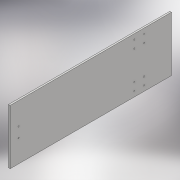
# Autodesk Inventor part: 内层17cm板
Saved by Autodesk Inventor 2017 (Build 210142000, 142)
## iProperties
Part Number: 内层17cm板
Material: 常规
Document SubType Name: 钣金
Designer: PANDA
Density: 1 g/cm^3
Sheet Metal Rule: 默认_mm
Appearance: 默认
Author: PANDA
Autodesk Inventor part; units mm, degrees
ref_plane "YZ Plane" through (0, 0, 0) normal (1, 0, 0) x (0, 1, 0)
ref_plane "XZ Plane" through (0, 0, 0) normal (0, 1, 0) x (-1, 0, 0)
ref_plane "XY Plane" through (0, 0, 0) normal (0, 0, 1) x (1, 0, 0)
sketch "草图8" plane through (0, 0, 0) normal (1, 0, 0) x (0, 1, 0)
  line L0 (250, 85) -> (-250, 85)
  line L1 (-250, 85) -> (-250, -85)
  line L2 (-250, -85) -> (250, -85)
  line L3 (250, -85) -> (250, 85)
  point P0 (0, 0)
  dimension "d22" = 500
  dimension "d23" = 170
  constraints: 8 end point, 2 parallel, 1 horizontal, 1 perpendicular
  measures "d22" distance of L2.end L1.end
  measures "d23" distance of L1.end L0.end
extrude "拉伸8" add sketch "草图8" along normal blind 5
sketch "草图9" plane through (5, 0, 0) normal (1, 0, 0) x (0, 0, -1)
  circle A0 centre (15.5, -224) radius 1.8
  point P0 (0, 0)
  dimension "d26" = 3.6
  constraints: 1 centre point
  measures "d26" diameter of A0
extrude "拉伸9" cut sketch "草图9" against normal through all
sketch "草图10" plane through (5, 0, 0) normal (1, 0, 0) x (0, 0, -1)
  circle A0 centre (-15.5, -224) radius 1.8
  point P0 (0, 0)
  dimension "d29" = 3.6
  constraints: 1 centre point
  measures "d29" diameter of A0
extrude "拉伸10" cut sketch "草图10" against normal through all
sketch "草图11" plane through (5, 0, 0) normal (1, 0, 0) x (0, 0, -1)
  circle A0 centre (-69, 165) radius 1.8
  point P0 (0, 0)
  dimension "d32" = 3.6
  constraints: 1 centre point
  measures "d32" diameter of A0
extrude "拉伸11" cut sketch "草图11" against normal through all
sketch "草图12" plane through (5, 0, 0) normal (1, 0, 0) x (0, 0, -1)
  circle A0 centre (69, 165) radius 1.8
  point P0 (0, 0)
  dimension "d35" = 3.6
  constraints: 1 centre point
  measures "d35" diameter of A0
extrude "拉伸12" cut sketch "草图12" against normal through all
sketch "草图13" plane through (5, 0, 0) normal (1, 0, 0) x (0, 0, -1)
  circle A0 centre (-45, 165) radius 1.8
  point P0 (0, 0)
  dimension "d38" = 3.6
  constraints: 1 centre point
  measures "d38" diameter of A0
extrude "拉伸13" cut sketch "草图13" against normal through all
sketch "草图14" plane through (5, 0, 0) normal (1, 0, 0) x (0, 0, -1)
  circle A0 centre (45, 165) radius 1.8
  point P0 (0, 0)
  dimension "d41" = 3.6
  constraints: 1 centre point
  measures "d41" diameter of A0
extrude "拉伸14" cut sketch "草图14" against normal through all
sketch "草图15" plane through (5, 0, 0) normal (1, 0, 0) x (0, 0, -1)
  circle A0 centre (-69, 135) radius 1.8
  point P0 (0, 0)
  dimension "d44" = 3.6
  constraints: 1 centre point
  measures "d44" diameter of A0
extrude "拉伸15" cut sketch "草图15" against normal through all
sketch "草图16" plane through (5, 0, 0) normal (1, 0, 0) x (0, 0, -1)
  circle A0 centre (-45, 135) radius 1.8
  point P0 (0, 0)
  dimension "d47" = 3.6
  constraints: 1 centre point
  measures "d47" diameter of A0
extrude "拉伸16" cut sketch "草图16" against normal through all
sketch "草图17" plane through (5, 0, 0) normal (1, 0, 0) x (0, 0, -1)
  circle A0 centre (45, 135) radius 1.8
  point P0 (0, 0)
  dimension "d50" = 3.6
  constraints: 1 centre point
  measures "d50" diameter of A0
extrude "拉伸17" cut sketch "草图17" against normal through all
sketch "草图18" plane through (5, 0, 0) normal (1, 0, 0) x (0, 0, -1)
  circle A0 centre (69, 135) radius 1.8
  point P0 (0, 0)
  dimension "d53" = 3.6
  constraints: 1 centre point
  measures "d53" diameter of A0
extrude "拉伸18" cut sketch "草图18" against normal through all
equation "\"折弯半径\" = 厚度"
equation "\"折弯释压宽度\" = 厚度"
equation "\"折弯释压深度\" = 0.5 * 厚度"
equation "\"拐角释压尺寸\" = 4 * 厚度"
equation "\"最小余量\" = 2 * 厚度"
equation "\"过渡半径\" = 折弯半径"
equation "\"Jacobi半径尺寸\" = 折弯半径"
equation "\"间隙大小\" = 厚度"
equation "\"厚度\" = 0.5"
